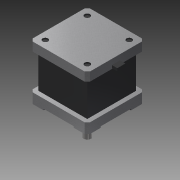
# Autodesk Inventor part: Stepper Motor NEMA 17
Saved by Autodesk Inventor 2014 SP1 (Build 180222100, 222)
## iProperties
Created: 2021-06-01
Part Number: Stepper Motor NEMA 17
Material: Rubber
Document SubType Name: Modeling
Designer: vivek
Density: 0.93 g/cm^3
Appearance: Rubber - Black - Version 1.1
Author: vivek
Autodesk Inventor part; units mm, degrees
ref_plane "YZ Plane" through (0, 0, 0) normal (1, 0, 0) x (0, 1, 0)
ref_plane "XZ Plane" through (0, 0, 0) normal (0, 1, 0) x (-1, 0, 0)
sketch "Sketch1" plane through (0, 0, 0) normal (0, 0, 1) x (1, 0, 0)
  line L0 (0, 0) -> (0, 3.4207)
  line L1 (0, 0) -> (9.2929, 0)
  line L2 (21.15, -21.15) -> (-21.15, -21.15)
  line L3 (-21.15, -21.15) -> (-21.15, 21.15)
  line L4 (-21.15, 21.15) -> (21.15, 21.15)
  line L5 (21.15, 21.15) -> (21.15, -21.15)
  point P0 (0, 21.15)
  point P1 (21.15, 0)
  dimension "d0" = 42.3
  dimension "d1" = 42.3
  constraints: 12 end point, 2 midpoint, 2 parallel, 2 perpendicular, 2 point on line, 1 horizontal, 1 vertical
  measures "d0" distance of L3.end L4.end
  measures "d1" distance of L2.end L3.end
extrude "Extrusion1" add sketch "Sketch1" along normal blind 39
sketch "Sketch2" plane through (0, 0, 0) normal (0, 0, -1) x (-1, 0, 0)
  line L0 (-21.15, 21.15) -> (-21.15, -21.15) projected
  circle A0 centre (-15.5, 15.5) radius 2
  circle A1 centre (15.5, 15.5) radius 2
  line L1 (-15.5, 15.5) -> (15.5, 15.5)
  line L2 (0, 0) -> (0, 5.3355)
  line L3 (0, 0) -> (5.467, 0)
  circle A2 centre (-15.5, -15.5) radius 2
  circle A3 centre (15.5, -15.5) radius 2
  line L4 (-15.5, -15.5) -> (15.5, -15.5)
  line L5 (-21.15, 21.15) -> (-11.15, 21.15)
  line L6 (-11.15, 21.15) -> (-11.15, 11.15)
  line L7 (-11.15, 11.15) -> (-21.15, 11.15)
  line L8 (-21.15, 11.15) -> (-21.15, 21.15)
  line L9 (21.15, 21.15) -> (11.15, 21.15)
  line L10 (11.15, 21.15) -> (11.15, 11.15)
  line L11 (11.15, 11.15) -> (21.15, 11.15)
  line L12 (21.15, 11.15) -> (21.15, 21.15)
  line L13 (21.15, -21.15) -> (11.15, -21.15)
  line L14 (11.15, -21.15) -> (11.15, -11.15)
  line L15 (11.15, -11.15) -> (21.15, -11.15)
  line L16 (21.15, -11.15) -> (21.15, -21.15)
  line L17 (-21.15, -21.15) -> (-11.15, -21.15)
  line L18 (-11.15, -21.15) -> (-11.15, -11.15)
  line L19 (-11.15, -11.15) -> (-21.15, -11.15)
  line L20 (-21.15, -11.15) -> (-21.15, -21.15)
  circle A4 centre (0, 0) radius 11
  point P0 (0, 15.5)
  point P1 (0, -15.5)
  dimension "d4" = 4
  dimension "d5" = 4
  dimension "d6" = 31
  dimension "d7" = 31
  dimension "d8" = 10
  dimension "d9" = 10
  dimension "d10" = 10
  dimension "d11" = 10
  dimension "d12" = 10
  dimension "d13" = 10
  dimension "d14" = 10
  dimension "d15" = 10
  dimension "d20" = 22
  constraints: 40 end point, 8 parallel, 7 perpendicular, 5 centre point, 4 horizontal, 3 symmetric about line, 1 coincident, 1 midpoint, 1 point on line, 2 other
  measures "d4" diameter of A0
  measures "d5" diameter of A1
  measures "d6" distance of L1.start L1.end
  measures "d7" distance of L4.start L1.start
  measures "d8" distance of L6.end L7.end
  measures "d9" distance of L5.end L6.end
  measures "d10" distance of L11.end L10.end
  measures "d11" distance of L10.end L9.end
  measures "d12" distance of L14.end L15.end
  measures "d13" distance of L13.end L14.end
  measures "d14" distance of L19.end L18.end
  measures "d15" distance of L18.end L17.end
  measures "d20" diameter of A4
extrude "Extrusion2" add sketch "Sketch2" along normal blind 1 contours A0 | L5 L6 L7 L0 | A1 | L10 L9 L12 L11 | A3 | L14 L15 L16 L13 | A2 | L19 L18 L17 L0
extrude "Extrusion3" cut sketch "Sketch2" along normal mid plane 2 contours A0 | A1 | A3 | A2
extrude "Extrusion4" add sketch "Sketch2" along normal blind 1 contours A4
fillet "Fillet1" radius 3 4 edges at (11.15, 11.15, -0.5) (11.15, -11.15, -0.5) (-11.15, -11.15, -0.5) (-11.15, 11.15, -0.5)
chamfer "Chamfer1" distance 2 angle 45 4 edges at (21.15, -21.15, 19) (-21.15, -21.15, 19) (-21.15, 21.15, 19) (21.15, 21.15, 19)
sketch "Sketch3" plane through (0, 0, -1) normal (0, 0, -1) x (-1, 0, 0)
  circle A0 centre (0, 0) radius 11 projected
  circle A1 centre (0, 0) radius 2.5
  dimension "d27" = 5
  constraints: 1 centre point, 1 coincident
  measures "d27" diameter of A1
extrude "Extrusion5" add sketch "Sketch3" along normal blind 22 contours A1
ref_plane "Work Plane1" through (0, 0, 19.5) normal (0, 0, 1) x (1, 0, 0)
mirror "Mirror1" about plane through (0, 0, 19.5) normal (0, 0, 1) of "Extrusion3"
sketch "Sketch4" plane through (21.15, -11.15, 0) normal (1, 0, 0) x (0, 0, -1)
  line L0 (-39, -8) -> (-39, 30.3) projected
  line L1 (-35, 14.15) -> (-33, 14.15)
  line L2 (-33, 14.15) -> (-33, 8.15)
  line L3 (-33, 8.15) -> (-35, 8.15)
  line L4 (-35, 8.15) -> (-35, 14.15)
  line L5 (-39, 11.15) -> (-36.6866, 11.15)
  point P0 (0, 11.15)
  point P1 (-35, 11.15)
  dimension "d31" = 2
  dimension "d32" = 6
  dimension "d33" = 4
  constraints: 10 end point, 2 midpoint, 2 parallel, 2 perpendicular, 1 horizontal, 1 point on line
  measures "d31" distance of L2.end L3.end
  measures "d32" distance of L1.end L2.end
  measures "d33" distance between parallel lines of L0 L4
extrude "Extrusion6" add sketch "Sketch4" along normal blind 4
sketch "Sketch6" plane through (0, 0, 19.5) normal (0, 0, 1) x (1, 0, 0)
  line L0 (-21.15, 19.15) -> (-19.15, 21.15) projected
  line L1 (-19.15, 21.15) -> (19.15, 21.15) projected
  line L2 (19.15, 21.15) -> (21.15, 19.15) projected
  line L3 (21.15, 19.15) -> (21.15, -19.15) projected
  line L4 (21.15, -19.15) -> (19.15, -21.15) projected
  line L5 (19.15, -21.15) -> (-19.15, -21.15) projected
  line L6 (-19.15, -21.15) -> (-21.15, -19.15) projected
  line L7 (-21.15, -19.15) -> (-21.15, 19.15) projected
  line L8 (-17.7379, 17.7408) -> (-17.7408, 17.7379)
  line L9 (-17.7408, -17.7379) -> (-17.7379, -17.7408)
  line L10 (17.7379, -17.7408) -> (17.7408, -17.7379)
  line L11 (17.7408, 17.7379) -> (17.7379, 17.7408)
  line L12 (-21.15, 14.9074) -> (-14.9074, 21.15)
  line L13 (-18.0287, 18.0287) -> (18.0287, 18.0287)
  line L14 (18.0287, 18.0287) -> (18.0287, -18.0287)
  line L15 (18.0287, -18.0287) -> (-18.0287, -18.0287)
  line L16 (-18.0287, -18.0287) -> (-18.0287, 18.0287)
  line L17 (-21.15, 14.9074) -> (-21.15, 19.15)
  line L18 (-19.15, 21.15) -> (-21.15, 19.15)
  line L19 (-19.15, 21.15) -> (-14.9074, 21.15)
  line L20 (-14.9074, -21.15) -> (-21.15, -14.9074)
  line L21 (-14.9074, -21.15) -> (-19.15, -21.15)
  line L22 (-21.15, -19.15) -> (-19.15, -21.15)
  line L23 (-21.15, -19.15) -> (-21.15, -14.9074)
  line L24 (21.15, -14.9074) -> (14.9074, -21.15)
  line L25 (21.15, -14.9074) -> (21.15, -19.15)
  line L26 (19.15, -21.15) -> (21.15, -19.15)
  line L27 (19.15, -21.15) -> (14.9074, -21.15)
  line L28 (14.9074, 21.15) -> (21.15, 14.9074)
  line L29 (14.9074, 21.15) -> (19.15, 21.15)
  line L30 (21.15, 19.15) -> (19.15, 21.15)
  line L31 (21.15, 19.15) -> (21.15, 14.9074)
  line L32 (-21.15, 14.9074) -> (-21.15, -14.9074)
  line L33 (-14.9074, -21.15) -> (14.9074, -21.15)
  line L34 (21.15, -14.9074) -> (21.15, 14.9074)
  line L35 (14.9074, 21.15) -> (-14.9074, 21.15)
  point P0 (0, 0)
  point P1 (18.0287, -18.0287)
  dimension "d43" = 3
  dimension "d46" = 360
  constraints: 56 end point, 6 collinear, 3 midpoint, 3 perpendicular, 2 parallel, 2 point on line, 1 horizontal, 37 other
  measures "d43" distance between parallel lines of L0 L12
extrude "Extrusion8" cut sketch "Sketch6" along normal mid plane 26 contours L0 L1 L12 L7 | L12 L16 L20 L7 | L1 L28 L13 L12 | L20 L5 L6 L7 | L1 L2 L3 L28 | L15 L24 L5 L20 | L28 L3 L24 L14 | L24 L3 L4 L5
body "Solid1"
